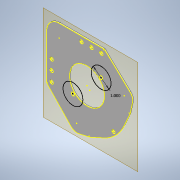
# Autodesk Inventor part: upper
Saved by Autodesk Inventor 2022 (Build 260153000, 153)
## iProperties
Created: 2022-03-17
Part Number: upper
Material: Generic
Document SubType Name: Modeling
Designer: zac-h
Density: 1 g/cm^3
Appearance: Default
Author: zac-h
Autodesk Inventor part; units mm, degrees
ref_plane "YZ Plane" through (0, 0, 0) normal (1, 0, 0) x (0, 1, 0)
ref_plane "XZ Plane" through (0, 0, 0) normal (0, 1, 0) x (-1, 0, 0)
ref_plane "XY Plane" through (0, 0, 0) normal (0, 0, 1) x (1, 0, 0)
ref_plane "Work Plane1" through (0, 0, 0) normal (0, 0, 1) x (1, 0, 0)
sketch "Sketch1" plane through (0, 0, 0) normal (0, 0, 1) x (1, 0, 0)
  line L0 (54.6745, 14.0094) -> (51.6007, 0.0667) projected
  arc A0 (54.6745, 14.0094) -> (51.7087, 23.6992) centre (44.6112, 16.228) ccw projected
  line L1 (19.1376, 54.6412) -> (51.7087, 23.6992) projected
  arc A1 (19.1376, 54.6412) -> (18.4488, 54.9162) centre (18.4488, 53.9162) ccw projected
  line L2 (-38.4967, 54.9162) -> (18.4488, 54.9162) projected
  arc A2 (-38.4967, 54.9162) -> (-54.9162, 38.4967) centre (-38.4967, 38.4967) ccw projected
  line L3 (-54.9162, -18.4488) -> (-54.9162, 38.4967) projected
  arc A3 (-54.9162, -18.4488) -> (-54.6412, -19.1376) centre (-53.9162, -18.4488) ccw projected
  line L4 (-23.6992, -51.7087) -> (-54.6412, -19.1376) projected
  arc A4 (-23.6992, -51.7087) -> (-14.0094, -54.6745) centre (-16.228, -44.6112) ccw projected
  line L5 (-0.0667, -51.6007) -> (-14.0094, -54.6745) projected
  arc A5 (-0.0667, -51.6007) -> (0.1266, -51.5369) centre (-0.282, -50.6241) ccw projected
  line L6 (17.6889, -43.6752) -> (0.1266, -51.5369) projected
  arc A6 (17.6889, -43.6752) -> (43.6752, -17.6889) centre (-3.3712, 3.3712) ccw projected
  line L7 (51.5369, -0.1266) -> (43.6752, -17.6889) projected
  arc A7 (51.5369, -0.1266) -> (51.6007, 0.0667) centre (50.6241, 0.282) ccw projected
  circle A8 centre (-3.3712, 3.3712) radius 39.37 projected
  circle A9 centre (-48.5312, 10.4312) radius 2.132 projected
  circle A10 centre (-48.5312, -2.2688) radius 2.132 projected
  circle A11 centre (-48.5312, -14.9688) radius 2.132 projected
  circle A12 centre (-10.4312, 48.5312) radius 2.132 projected
  circle A13 centre (2.2688, 48.5312) radius 2.132 projected
  circle A14 centre (14.9688, 48.5312) radius 2.132 projected
  circle A15 centre (30.3259, -30.3259) radius 2.132 projected
  circle A16 centre (-3.3712, 3.3712) radius 22.225
  line L8 (-3.3712, 3.3712) -> (14.5893, 21.3317) construction
  line L9 (-3.3712, 3.3712) -> (22.0288, 3.3712) construction
  circle A17 centre (14.5893, 21.3317) radius 2.132
  circle A18 centre (-21.3317, -14.5893) radius 2.132
  point P0 (0, 0)
  dimension "d0" = 44.45
  dimension "d1" = 25.4
  dimension "d2" = 45
  dimension "d3" = 4.264
  dimension "d6" = 360
  constraints: 4 end point, 3 centre point, 2 coincident, 1 equal length, 1 horizontal, 5 other
  measures "d0" diameter of A16
  measures "d1" distance of L8.start L8.end
  measures "d2" angle of L9 L8
  measures "d3" diameter of A17
extrude "Extrusion1" add sketch "Sketch1" along normal blind 1.2 contours L0 A7 L7 A6 L6 A5 L5 A4 L4 A3 L3 A2 L2 A1 L1 A0 | A8
sketch "Sketch2" plane through (0, 0, 1.2) normal (0, 0, 1) x (1, 0, 0)
  line L0 (18.4488, 54.9162) -> (-38.4967, 54.9162) projected
  arc A0 (-38.4967, 54.9162) -> (-54.9162, 38.4967) centre (-38.4967, 38.4967) ccw projected
  line L1 (-54.9162, 38.4967) -> (-54.9162, -18.4488) projected
  arc A1 (-54.9162, -18.4488) -> (-54.6412, -19.1376) centre (-53.9162, -18.4488) ccw projected
  line L2 (-54.6412, -19.1376) -> (-23.6992, -51.7087) projected
  arc A2 (-23.6992, -51.7087) -> (-14.0094, -54.6745) centre (-16.228, -44.6112) ccw projected
  line L3 (-14.0094, -54.6745) -> (-0.0667, -51.6007) projected
  arc A3 (-0.0667, -51.6007) -> (0.1266, -51.5369) centre (-0.282, -50.6241) ccw projected
  line L4 (0.1266, -51.5369) -> (17.6889, -43.6752) projected
  arc A4 (17.6889, -43.6752) -> (43.6752, -17.6889) centre (-3.3712, 3.3712) ccw projected
  line L5 (43.6752, -17.6889) -> (51.5369, -0.1266) projected
  arc A5 (51.5369, -0.1266) -> (51.6007, 0.0667) centre (50.6241, 0.282) ccw projected
  line L6 (51.6007, 0.0667) -> (54.6745, 14.0094) projected
  arc A6 (54.6745, 14.0094) -> (51.7087, 23.6992) centre (44.6112, 16.228) ccw projected
  line L7 (51.7087, 23.6992) -> (19.1376, 54.6412) projected
  arc A7 (19.1376, 54.6412) -> (18.4488, 54.9162) centre (18.4488, 53.9162) ccw projected
  circle A8 centre (30.3259, -30.3259) radius 2.132 projected
  circle A9 centre (14.9688, 48.5312) radius 2.132 projected
  circle A10 centre (2.2688, 48.5312) radius 2.132 projected
  circle A11 centre (-10.4312, 48.5312) radius 2.132 projected
  circle A12 centre (-48.5312, -14.9688) radius 2.132 projected
  circle A13 centre (-48.5312, -2.2688) radius 2.132 projected
  circle A14 centre (-48.5312, 10.4312) radius 2.132 projected
  circle A15 centre (-21.3317, -14.5893) radius 2.132 projected
  circle A16 centre (14.5893, 21.3317) radius 2.132 projected
  circle A17 centre (-3.3712, 3.3712) radius 22.225 projected
  circle A18 centre (14.5893, 21.3317) radius 2.132 projected
  circle A19 centre (14.5893, 21.3317) radius 12.7
  circle A20 centre (-21.3317, -14.5893) radius 12.7
  point P0 (0, 0)
  dimension "d10" = 25.4
  constraints: 2 centre point, 2 coincident, 1 equal radius
  measures "d10" diameter of A19
body "Solid1"
